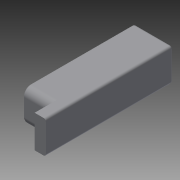
# Autodesk Inventor part: Flight Battery 5000 mah 5S
Saved by Autodesk Inventor 2015 (Build 190159000, 159)
## iProperties
Created: 2018-07-21
Part Number: Flight Battery 5000 mah 5S
Material: Generic
Document SubType Name: Modeling
Designer: Michael Gunderman
Mass: 542 g
Surface Area: 325.67 cm^2
Volume: 326.07 cm^3
Density: 1.66222 g/cm^3
Appearance: Default
Author: Michael Gunderman
Autodesk Inventor part; units mm, degrees
ref_plane "YZ Plane" through (0, 0, 0) normal (1, 0, 0) x (0, 1, 0)
ref_plane "XZ Plane" through (0, 0, 0) normal (0, 1, 0) x (-1, 0, 0)
ref_plane "XY Plane" through (0, 0, 0) normal (0, 0, 1) x (1, 0, 0)
sketch "Sketch1" plane through (0, 0, 0) normal (0, 1, 0) x (-1, 0, 0)
  line L0 (14.6941, 0) -> (51, 0)
  line L1 (51, 0) -> (51, -146)
  line L2 (51, -146) -> (0, -146)
  line L3 (0, -146) -> (0, 0)
  line L4 (14.6941, 0) -> (14.6941, 20.4717)
  line L5 (14.6941, 20.4717) -> (0, 20.4717)
  line L6 (0, 20.4717) -> (0, 0)
  dimension "d0" = 51
  dimension "d1" = 146
  constraints: 14 end point, 4 perpendicular, 2 parallel, 1 horizontal
  measures "d0" distance of L1.end L2.end
  measures "d1" distance of L0.end L1.end
extrude "Extrusion1" add sketch "Sketch1" along normal blind 42.5
fillet "Fillet1" radius 10 2 edges at (-32.847, 42.5, 0) (-32.847, 0, 0)
fillet "Fillet2" radius 3 11 edges at (-51, 2.9289, -2.9289) (-51, 21.25, 0) (-51, 39.5711, -2.9289) (-51, 42.5, -78) (-51, 0, -78) (-51, 21.25, -146) (-25.5, 0, -146) (0, 21.25, -146) (0, 0, -73) (0, 42.5, -73) (-25.5, 42.5, -146)
body "Solid1"
